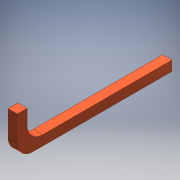
# Autodesk Inventor part: pins
Saved by Autodesk Inventor 2016 (Build 200138000, 138)
## iProperties
Created: 2016-07-25
Part Number: pins
Material: Copper
Document SubType Name: Modeling
Designer: Jonathan
Density: 8.94 g/cm^3
Appearance: Copper - Satin
Author: Jonathan
Autodesk Inventor part; units mm, degrees
ref_plane "YZ Plane" through (0, 0, 0) normal (1, 0, 0) x (0, 1, 0)
ref_plane "XZ Plane" through (0, 0, 0) normal (0, 1, 0) x (-1, 0, 0)
ref_plane "XY Plane" through (0, 0, 0) normal (0, 0, 1) x (1, 0, 0)
sketch "Sketch1" plane through (0, 0, 0) normal (1, 0, 0) x (0, 1, 0)
  line L0 (-9.36, 2.62) -> (-9.36, 0.64)
  line L1 (-9.36, 0.64) -> (0, 0.64)
  line L2 (0, 0.64) -> (0, 0)
  line L3 (0, 0) -> (-10, 0)
  line L4 (-10, 0) -> (-10, 2.62)
  line L5 (-10, 2.62) -> (-9.36, 2.62)
  point P0 (0, 0.32)
  dimension "d0" = 0.64
  dimension "d1" = 0.64
  dimension "d2" = 2.3
  dimension "d3" = 10
  constraints: 12 end point, 5 perpendicular, 1 coincident, 1 midpoint, 1 vertical
  measures "d0" distance between parallel lines of L3 L1
  measures "d1" distance between parallel lines of L4 L0
  measures "d2" distance from line of L5 point (0, 0.32)
  measures "d3" distance between parallel lines of L4 L2
extrude "Extrusion1" add sketch "Sketch1" along normal mid plane 0.6
fillet "Fillet1" radius 1 2 edges at (0, -9.36, 0.64) (0, -10, 0)
body "Solid1"
